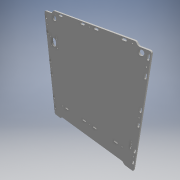
# Autodesk Inventor part: painel esquerdo
Saved by Autodesk Inventor 2016 (Build 200138000, 138)
## iProperties
Created: 2016-08-08
Part Number: painel esquerdo
Material: Generic
Document SubType Name: Modeling
Designer: Waldo
Density: 1 g/cm^3
Appearance: Default
Author: Waldo
Autodesk Inventor part; units mm, degrees
ref_plane "YZ Plane" through (0, 0, 0) normal (1, 0, 0) x (0, 1, 0)
ref_plane "XZ Plane" through (0, 0, 0) normal (0, 1, 0) x (-1, 0, 0)
ref_plane "XY Plane" through (0, 0, 0) normal (0, 0, 1) x (1, 0, 0)
sketch "Sketch1" plane through (0, 0, 0) normal (0, 1, 0) x (-1, 0, 0)
  line L0 (-184.1567, -90.0562) -> (-184.1567, -118.0908)
  line L1 (-188.2438, -118.0908) -> (-188.2438, -90.0562)
  line L2 (173.9968, 182.2069) -> (173.9968, 192.2069)
  line L3 (167.7968, 192.2069) -> (167.7968, 182.2069)
  line L4 (14.5968, -131.4908) -> (4.5968, -131.4908)
  line L5 (4.5968, -137.6908) -> (14.5968, -137.6908)
  line L6 (105.0968, -131.4908) -> (95.0968, -131.4908)
  line L7 (95.0968, -137.6908) -> (105.0968, -137.6908)
  line L8 (-135.9032, -137.6908) -> (-125.9032, -137.6908)
  line L9 (-125.9032, -131.4908) -> (-135.9032, -131.4908)
  line L10 (-45.4032, -137.6908) -> (-35.4032, -137.6908)
  line L11 (-35.4032, -131.4908) -> (-45.4032, -131.4908)
  line L12 (14.5968, 210.5092) -> (4.5968, 210.5092)
  line L13 (4.5968, 204.3092) -> (14.5968, 204.3092)
  line L14 (105.0968, 210.5092) -> (95.0968, 210.5092)
  line L15 (95.0968, 204.3092) -> (105.0968, 204.3092)
  line L16 (-135.9032, 204.3092) -> (-125.9032, 204.3092)
  line L17 (-125.9032, 210.5092) -> (-135.9032, 210.5092)
  line L18 (-45.4032, 204.3092) -> (-35.4032, 204.3092)
  line L19 (-35.4032, 210.5092) -> (-45.4032, 210.5092)
  line L20 (173.9968, 132.2069) -> (173.9968, 142.2069)
  line L21 (167.7968, 142.2069) -> (167.7968, 132.2069)
  line L22 (173.9968, 29.7671) -> (173.9968, 39.7671)
  line L23 (167.7968, 39.7671) -> (167.7968, 29.7671)
  line L24 (173.9968, -21.9484) -> (173.9968, -11.9484)
  line L25 (167.7968, -11.9484) -> (167.7968, -21.9484)
  line L26 (173.9968, -124.3882) -> (173.9968, -114.3882)
  line L27 (167.7968, -114.3882) -> (167.7968, -124.3882)
  line L28 (173.9968, -174.3882) -> (173.9968, -164.3882)
  line L29 (167.7968, -164.3882) -> (167.7968, -174.3882)
  line L30 (-204.8032, -11.9484) -> (-204.8032, -21.9484)
  line L31 (-198.6032, -21.9484) -> (-198.6032, -11.9484)
  line L32 (-204.8032, 39.7671) -> (-204.8032, 29.7671)
  line L33 (-198.6032, 29.7671) -> (-198.6032, 39.7671)
  line L34 (-204.8032, -164.3882) -> (-204.8032, -174.3882)
  line L35 (-198.6032, -174.3882) -> (-198.6032, -164.3882)
  line L36 (-204.8032, -114.3882) -> (-204.8032, -124.3882)
  line L37 (-198.6032, -124.3882) -> (-198.6032, -114.3882)
  line L38 (-204.8032, 142.2069) -> (-204.8032, 132.2069)
  line L39 (-198.6032, 132.2069) -> (-198.6032, 142.2069)
  line L40 (-204.8032, 192.2069) -> (-204.8032, 182.2069)
  line L41 (-198.6032, 182.2069) -> (-198.6032, 192.2069)
  line L42 (132.2968, 115.5069) -> (132.2968, 107.0069)
  line L43 (154.2968, 107.0069) -> (154.2968, 115.5069)
  line L44 (160.5968, 94.4092) -> (160.5968, 102.9092)
  line L45 (157.3968, 102.9092) -> (157.3968, 94.4092)
  line L46 (129.5968, 125.4092) -> (129.5968, 133.9092)
  line L47 (126.3968, 133.9092) -> (126.3968, 125.4092)
  line L48 (135.2533, -199.1268) -> (138.549, -203.0545)
  line L49 (145.0604, -206.0908) -> (171.0968, -206.0908)
  line L50 (177.0968, -200.0908) -> (177.0968, 198.0069)
  line L51 (171.0968, 204.0069) -> (145.0968, 204.0069)
  line L52 (138.5854, 207.0432) -> (135.3719, 210.8729)
  line L53 (128.8605, 213.9092) -> (-159.667, 213.9092)
  line L54 (-166.1784, 210.8729) -> (-169.3918, 207.0432)
  line L55 (-175.9032, 204.0069) -> (-201.9032, 204.0069)
  line L56 (-207.9032, 198.0069) -> (-207.9032, -200.0908)
  line L57 (-201.9032, -206.0908) -> (-175.8668, -206.0908)
  line L58 (-169.3555, -203.0545) -> (-166.0597, -199.1268)
  line L59 (-159.5483, -196.0905) -> (128.7419, -196.0905)
  line L60 (160.5968, 125.4092) -> (160.5968, 133.9092)
  line L61 (157.3968, 133.9092) -> (157.3968, 125.4092)
  line L62 (129.5968, 94.4092) -> (129.5968, 102.9092)
  line L63 (126.3968, 102.9092) -> (126.3968, 94.4092)
  arc A0 (-188.2438, -118.0908) -> (-184.1567, -118.0908) centre (-186.2002, -118.0908) ccw
  arc A1 (-184.1567, -90.0562) -> (-188.2438, -90.0562) centre (-186.2002, -90.0562) ccw
  arc A2 (167.7968, 182.2069) -> (173.9968, 182.2069) centre (170.8968, 182.2069) ccw
  arc A3 (173.9968, 192.2069) -> (167.7968, 192.2069) centre (170.8968, 192.2069) ccw
  arc A4 (14.5968, -137.6908) -> (14.5968, -131.4908) centre (14.5968, -134.5908) ccw
  arc A5 (4.5968, -131.4908) -> (4.5968, -137.6908) centre (4.5968, -134.5908) ccw
  arc A6 (105.0968, -137.6908) -> (105.0968, -131.4908) centre (105.0968, -134.5908) ccw
  arc A7 (95.0968, -131.4908) -> (95.0968, -137.6908) centre (95.0968, -134.5908) ccw
  arc A8 (-135.9032, -131.4908) -> (-135.9032, -137.6908) centre (-135.9032, -134.5908) ccw
  arc A9 (-125.9032, -137.6908) -> (-125.9032, -131.4908) centre (-125.9032, -134.5908) ccw
  arc A10 (-45.4032, -131.4908) -> (-45.4032, -137.6908) centre (-45.4032, -134.5908) ccw
  arc A11 (-35.4032, -137.6908) -> (-35.4032, -131.4908) centre (-35.4032, -134.5908) ccw
  arc A12 (14.5968, 204.3092) -> (14.5968, 210.5092) centre (14.5968, 207.4092) ccw
  arc A13 (4.5968, 210.5092) -> (4.5968, 204.3092) centre (4.5968, 207.4092) ccw
  arc A14 (105.0968, 204.3092) -> (105.0968, 210.5092) centre (105.0968, 207.4092) ccw
  arc A15 (95.0968, 210.5092) -> (95.0968, 204.3092) centre (95.0968, 207.4092) ccw
  arc A16 (-135.9032, 210.5092) -> (-135.9032, 204.3092) centre (-135.9032, 207.4092) ccw
  arc A17 (-125.9032, 204.3092) -> (-125.9032, 210.5092) centre (-125.9032, 207.4092) ccw
  arc A18 (-45.4032, 210.5092) -> (-45.4032, 204.3092) centre (-45.4032, 207.4092) ccw
  arc A19 (-35.4032, 204.3092) -> (-35.4032, 210.5092) centre (-35.4032, 207.4092) ccw
  arc A20 (167.7968, 132.2069) -> (173.9968, 132.2069) centre (170.8968, 132.2069) ccw
  arc A21 (173.9968, 142.2069) -> (167.7968, 142.2069) centre (170.8968, 142.2069) ccw
  arc A22 (167.7968, 29.7671) -> (173.9968, 29.7671) centre (170.8968, 29.7671) ccw
  arc A23 (173.9968, 39.7671) -> (167.7968, 39.7671) centre (170.8968, 39.7671) ccw
  arc A24 (167.7968, -21.9484) -> (173.9968, -21.9484) centre (170.8968, -21.9484) ccw
  arc A25 (173.9968, -11.9484) -> (167.7968, -11.9484) centre (170.8968, -11.9484) ccw
  arc A26 (167.7968, -124.3882) -> (173.9968, -124.3882) centre (170.8968, -124.3882) ccw
  arc A27 (173.9968, -114.3882) -> (167.7968, -114.3882) centre (170.8968, -114.3882) ccw
  arc A28 (167.7968, -174.3882) -> (173.9968, -174.3882) centre (170.8968, -174.3882) ccw
  arc A29 (173.9968, -164.3882) -> (167.7968, -164.3882) centre (170.8968, -164.3882) ccw
  arc A30 (-198.6032, -11.9484) -> (-204.8032, -11.9484) centre (-201.7032, -11.9484) ccw
  arc A31 (-204.8032, -21.9484) -> (-198.6032, -21.9484) centre (-201.7032, -21.9484) ccw
  arc A32 (-198.6032, 39.7671) -> (-204.8032, 39.7671) centre (-201.7032, 39.7671) ccw
  arc A33 (-204.8032, 29.7671) -> (-198.6032, 29.7671) centre (-201.7032, 29.7671) ccw
  arc A34 (-198.6032, -164.3882) -> (-204.8032, -164.3882) centre (-201.7032, -164.3882) ccw
  arc A35 (-204.8032, -174.3882) -> (-198.6032, -174.3882) centre (-201.7032, -174.3882) ccw
  arc A36 (-198.6032, -114.3882) -> (-204.8032, -114.3882) centre (-201.7032, -114.3882) ccw
  arc A37 (-204.8032, -124.3882) -> (-198.6032, -124.3882) centre (-201.7032, -124.3882) ccw
  arc A38 (-198.6032, 142.2069) -> (-204.8032, 142.2069) centre (-201.7032, 142.2069) ccw
  arc A39 (-204.8032, 132.2069) -> (-198.6032, 132.2069) centre (-201.7032, 132.2069) ccw
  arc A40 (-198.6032, 192.2069) -> (-204.8032, 192.2069) centre (-201.7032, 192.2069) ccw
  arc A41 (-204.8032, 182.2069) -> (-198.6032, 182.2069) centre (-201.7032, 182.2069) ccw
  arc A42 (154.2968, 115.5069) -> (132.2968, 115.5069) centre (143.2968, 115.5069) ccw
  arc A43 (132.2968, 107.0069) -> (154.2968, 107.0069) centre (143.2968, 107.0069) ccw
  circle A44 centre (129.7968, 191.5069) radius 8
  circle A45 centre (-182.3032, 191.5069) radius 8
  arc A46 (160.5968, 102.9092) -> (157.3968, 102.9092) centre (158.9968, 102.9092) ccw
  arc A47 (157.3968, 94.4092) -> (160.5968, 94.4092) centre (158.9968, 94.4092) ccw
  arc A48 (129.5968, 133.9092) -> (126.3968, 133.9092) centre (127.9968, 133.9092) ccw
  arc A49 (126.3968, 125.4092) -> (129.5968, 125.4092) centre (127.9968, 125.4092) ccw
  arc A50 (135.2533, -199.1268) -> (128.7419, -196.0905) centre (128.7419, -204.5905) ccw
  arc A51 (138.549, -203.0545) -> (145.0604, -206.0908) centre (145.0604, -197.5908) ccw
  arc A52 (171.0968, -206.0908) -> (177.0968, -200.0908) centre (171.0968, -200.0908) ccw
  arc A53 (177.0968, 198.0069) -> (171.0968, 204.0069) centre (171.0968, 198.0069) ccw
  arc A54 (138.5854, 207.0432) -> (145.0968, 204.0069) centre (145.0968, 212.5069) ccw
  arc A55 (135.3719, 210.8729) -> (128.8605, 213.9092) centre (128.8605, 205.4092) ccw
  arc A56 (-159.667, 213.9092) -> (-166.1784, 210.8729) centre (-159.667, 205.4092) ccw
  arc A57 (-175.9032, 204.0069) -> (-169.3918, 207.0432) centre (-175.9032, 212.5069) ccw
  arc A58 (-201.9032, 204.0069) -> (-207.9032, 198.0069) centre (-201.9032, 198.0069) ccw
  arc A59 (-207.9032, -200.0908) -> (-201.9032, -206.0908) centre (-201.9032, -200.0908) ccw
  arc A60 (-175.8668, -206.0908) -> (-169.3555, -203.0545) centre (-175.8668, -197.5908) ccw
  arc A61 (-159.5483, -196.0905) -> (-166.0597, -199.1268) centre (-159.5483, -204.5905) ccw
  circle A62 centre (-15.4032, 205.9092) radius 1.55
  arc A63 (160.5968, 133.9092) -> (157.3968, 133.9092) centre (158.9968, 133.9092) ccw
  arc A64 (157.3968, 125.4092) -> (160.5968, 125.4092) centre (158.9968, 125.4092) ccw
  arc A65 (129.5968, 102.9092) -> (126.3968, 102.9092) centre (127.9968, 102.9092) ccw
  arc A66 (126.3968, 94.4092) -> (129.5968, 94.4092) centre (127.9968, 94.4092) ccw
  circle A67 centre (125.0968, 205.9092) radius 1.55
  circle A68 centre (-155.9032, 205.9092) radius 1.55
  circle A69 centre (-15.4032, -136.0908) radius 1.55
  circle A70 centre (125.0968, -136.0908) radius 1.55
  circle A71 centre (-155.9032, -136.0908) radius 1.55
  circle A72 centre (-200.1532, 162.2069) radius 1.6
  circle A73 centre (-200.1532, 8.9094) radius 1.6
  circle A74 centre (-200.1532, -144.3882) radius 1.6
  circle A75 centre (169.3468, -144.3882) radius 1.6
  circle A76 centre (169.3468, 8.9094) radius 1.6
  circle A77 centre (169.3468, 162.2069) radius 1.6
  circle A78 centre (-182.3032, 191.5069) radius 4
  circle A79 centre (129.7968, 191.5069) radius 4
  point P0 (0, 0)
  constraints: 190 tangent, 128 end point, 128 point on circle, 80 centre point, 28 parallel, 27 equal radius, 8 perpendicular, 1 collinear
extrude "Extrusion1" add sketch "Sketch1" along normal blind 6 contours A50 L59 A61 L58 A60 L57 A59 L56 A58 L55 A57 L54 A56 L53 A55 L52 A54 L51 A53 L50 A52 L49 A51 L48
body "Solid1"
